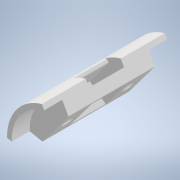
# Autodesk Inventor part: camera fixator
Saved by Autodesk Inventor 2022 (Build 260153000, 153)
## iProperties
Created: 2024-10-14
Part Number: camera fixator
Material: Типовые
Document SubType Name: Modeling
Designer: Andrey
Density: 1 g/cm^3
Appearance: По умолчанию
Author: Andrey
Autodesk Inventor part; units mm, degrees
ref_plane "YZ Plane" through (0, 0, 0) normal (1, 0, 0) x (0, 1, 0)
ref_plane "XZ Plane" through (0, 0, 0) normal (0, 1, 0) x (-1, 0, 0)
ref_plane "XY Plane" through (0, 0, 0) normal (0, 0, 1) x (1, 0, 0)
sketch "Эскиз1" plane through (0, 0, 0) normal (0, 0, 1) x (1, 0, 0)
  arc A0 (1.1623, 11.7426) -> (-10.9422, -4.4168) centre (0, 0) ccw projected
  line L0 (1.1623, 11.7426) -> (-10.9422, -4.4168) projected
  line L1 (-10.9422, -4.4168) -> (-12.1072, -5.9721) projected
  arc A1 (1.1623, 11.7426) -> (-10.9422, -4.4168) centre (0, 0) ccw projected
  line L2 (2.8533, 14) -> (1.1623, 11.7426) projected
  arc A2 (-8.1467, 10.7648) -> (-12.1072, -5.9721) centre (0, 0) ccw projected
  circle A3 centre (0, 0) radius 13.5
  circle A4 centre (0, 0) radius 11.8
  circle A5 centre (0, 0) radius 13.3
  circle A6 centre (0, 0) radius 12
  line L3 (-8.1467, 14) -> (2.8533, 14) projected
  line L4 (-8.1467, 14) -> (-8.1467, 10.7648) projected
  point P0 (2.3273, 13.2979)
  point P1 (-11.0819, -4.6034)
  point P2 (1.302, 11.9292)
  point P3 (2.1926, 13.118)
  point P4 (-11.9725, -5.7923)
  dimension "d1" = 0.2
  dimension "d2" = 0.2
  constraints: 2 centre point, 1 coincident, 6 other
extrude "Выдавливание1" add sketch "Эскиз1" along normal mid plane 34 contours A6 L1 A5 L2 picked at (-9.9488, 8.0267)
sketch "Эскиз2" plane through (0, 0, 0) normal (0, 0, 1) x (1, 0, 0)
  arc A0 (1.1623, 11.7426) -> (-10.9422, -4.4168) centre (0, 0) ccw projected
  line L0 (1.1623, 11.7426) -> (-10.9422, -4.4168) projected
  arc A1 (1.302, 11.9292) -> (-11.0819, -4.6034) centre (0, 0) ccw projected
  line L1 (-14.5944, -9.2926) -> (2.8533, 14) projected
extrude "Выдавливание2" add sketch "Эскиз2" along normal mid plane 24
sketch "Эскиз3" plane through (0, 0, 0) normal (0, 0, 1) x (1, 0, 0)
  arc A0 (1.302, 11.9292) -> (-11.0819, -4.6034) centre (0, 0) ccw projected
  line L0 (-11.0819, -4.6034) -> (1.302, 11.9292) projected
  arc A1 (2.1926, 13.118) -> (-11.9725, -5.7923) centre (0, 0) ccw projected
  arc A2 (-8.1467, 10.7648) -> (-12.1072, -5.9721) centre (0, 0) ccw projected
  line L1 (1.302, 11.9292) -> (-11.0819, -4.6034) projected
  line L2 (-4.8899, 3.6629) -> (-10.8048, 8.0935)
  line L3 (-10.8048, 8.0935) -> (-8.8039, 6.5947)
  line L4 (-11.3519, 3.1932) -> (-6.256, 9.9963)
  line L5 (-6.256, 9.9963) -> (-2.2942, 7.0286)
  line L6 (-2.2942, 7.0286) -> (-7.3901, 0.2256)
  line L7 (-7.3901, 0.2256) -> (-11.3519, 3.1932)
  line L8 (-12.1918, 3.0727) -> (-6.3765, 10.8362)
  line L9 (-6.3765, 10.8362) -> (-1.4543, 7.1491)
  line L10 (-1.4543, 7.1491) -> (-7.2696, -0.6143)
  line L11 (-7.2696, -0.6143) -> (-12.1918, 3.0727)
  point P0 (-4.8422, 3.6271)
  dimension "d7" = 2.5
  dimension "d8" = 8.5
  dimension "d9" = 4.95
  dimension "d12" = 0.6
  dimension "d13" = 9.7
  constraints: 20 end point, 7 perpendicular, 3 midpoint, 2 point on line, 1 point on circle, 3 other
  measures "d7" distance of L3.end L2.end
  measures "d8" distance of L4.start L4.end
  measures "d9" distance of L4.end L5.end
  measures "d12" distance between parallel lines of L7 L11
  measures "d13" distance between parallel lines of L9 L11
extrude "Выдавливание3" cut sketch "Эскиз3" along normal mid plane 9.7 contours L9 L0 L5 L4 L2 L8 A0 | A0 L8 L9 | L9 L10 L11 L0 L7 L6 L5 | L5 L6 L7 L0 | L0 L2 L4 L5 | L2 L4 L7 L0 L11 A0 L8 | L0 L7 L4 L2 | A0 L11 L8
sketch "Эскиз4" plane through (-1.9823, 7.5446, -4.85) normal (-0.5995217, -0.8003585, 0) x (0.8003585, -0.5995217, 0)
  line L0 (0, 9.7) -> (0, 0) projected
  line L1 (0, 9.7) -> (-5.4903, 9.7) projected
  line L2 (-5.4903, 0) -> (-5.4903, 9.7) projected
  line L3 (-5.4903, 0) -> (0, 0) projected
  line L4 (-5.4903, 9.7) -> (-2.7452, 9.7)
  line L5 (-2.7452, 0) -> (-2.7452, 9.7)
  point P0 (6.1097, 4.85)
  constraints: 4 end point, 2 midpoint, 1 perpendicular
extrude "Выдавливание4" cut sketch "Эскиз4" against normal blind 9.7 contours L5 L3 L2 L1
fillet "Сопряжение1" radius 0.6 3 edges at (-5.3836, 12.1617, 0) (-4.1794, 9.1904, 0) (-1.1375, 13.2513, 0)
sketch "Эскиз5" plane through (0, 0, 17) normal (0, 0, 1) x (1, 0, 0)
  arc A0 (2.1926, 13.118) -> (-11.9725, -5.7923) centre (0, 0) ccw projected
  circle A1 centre (0, 0) radius 13.3
  line L0 (2.8533, 17.048) -> (2.8533, 14) projected
  circle A2 centre (0, 0) radius 2.8533
  line L1 (9.8804, -12.4095) -> (-5.8229, 16.921)
  line L2 (0, 0) -> (2.5154, 1.3467)
  line L3 (-19.8346, 1.2413) -> (17.8745, -6.661)
  line L4 (0, 0) -> (-0.5852, -2.7926)
  line L5 (0, 0) -> (-4.8899, 3.6629)
  line L6 (-1.9823, 7.5446) -> (-7.7976, -0.2189) projected
  point P0 (5.4035, -4.0476)
  point P1 (-13.2994, -0.1282)
  point P2 (-11.9725, -5.7923)
  point P3 (8.6469, -10.1055)
  point P4 (12.1289, -5.457)
  point P5 (-3.6161, 12.799)
  dimension "d19" = 115
  dimension "d20" = 115
  constraints: 10 end point, 2 coincident, 2 point on circle, 2 point on line, 2 tangent, 1 centre point, 1 midpoint, 1 perpendicular, 3 other
  measures "d19" angle of L4 L5
  measures "d20" angle of L2 L5
extrude "Выдавливание5" cut sketch "Эскиз5" against normal blind 40 contours A1 L3 L1 A0 | L3 L1 A1 A0
sketch "Эскиз6" plane through (-8.4854, -1.137, 12) normal (0.8003585, -0.5995217, 0) x (0, 0, -1)
  line L0 (0, 0) -> (24, 0) projected
  line L1 (24, 11.9944) -> (24, 0) projected
  line L2 (24, 11.9944) -> (0, 11.9944) projected
  line L3 (0, 0) -> (0, 11.9944) projected
  line L4 (16.85, 10.8472) -> (16.85, 1.1472) projected
  line L5 (16.85, 1.1472) -> (7.15, 1.1472) projected
  line L6 (7.15, 1.1472) -> (7.15, 10.8472) projected
  line L7 (7.15, 10.8472) -> (16.85, 10.8472) projected
  line L8 (0, 0) -> (0, 11.9944) projected
  line L9 (0, 5.9972) -> (7.15, 5.9972)
  line L10 (7.15, 1.1472) -> (7.15, 10.8472) projected
  line L11 (16.85, 1.1472) -> (16.85, 9.5257) projected
  line L12 (16.85, 5.9972) -> (24, 5.9972)
  circle A0 centre (3.575, 5.9972) radius 1.6
  circle A1 centre (20.425, 5.9972) radius 1.6
  point P0 (12, 5.9972)
  dimension "d23" = 3.2
  dimension "d24" = 3.2
  constraints: 5 midpoint, 4 end point, 2 centre point, 2 point on line
  measures "d23" diameter of A0
  measures "d24" diameter of A1
extrude "Выдавливание6" cut sketch "Эскиз6" against normal blind 40 contours A0 L9 | L9 A0 | A1 L12 | L12 A1
